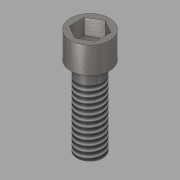
# Autodesk Inventor part: Bolt 2.0
Saved by Autodesk Inventor 2017 (Build 210142000, 142)
## iProperties
Created: 2017-01-01
Part Number: Bolt 2.0
Material: Steel, Galvanized
Document SubType Name: Modeling
Designer: qupec
Density: 7.85 g/cm^3
Appearance: Galvanized
Author: qupec
Autodesk Inventor part; units mm, degrees
ref_plane "YZ Plane" through (0, 0, 0) normal (1, 0, 0) x (0, 1, 0)
ref_plane "XZ Plane" through (0, 0, 0) normal (0, 1, 0) x (-1, 0, 0)
ref_plane "XY Plane" through (0, 0, 0) normal (0, 0, 1) x (1, 0, 0)
sketch "Sketch1" plane through (0, 0, 0) normal (0, 1, 0) x (-1, 0, 0)
  circle A0 centre (0, 0) radius 3.1369
  dimension "d0" = 6.2738
  constraints: 1 centre point, 1 coincident
  measures "d0" diameter of A0
extrude "Extrusion1" add sketch "Sketch1" along normal mid plane 6.35
sketch "Sketch2" plane through (0, 3.175, 0) normal (0, 1, 0) x (1, 0, 0)
  circle A0 centre (0, 0) radius 4.699
  dimension "d3" = 9.398
  constraints: 1 centre point, 1 coincident
  measures "d3" diameter of A0
extrude "Extrusion2" add sketch "Sketch2" along normal blind 6.35
sketch "Sketch3" plane through (0, -3.175, 0) normal (0, -1, 0) x (1, 0, 0)
  circle A0 centre (0, 0) radius 3.1369
  constraints: 1 centre point, 1 coincident
extrude "Extrusion3" add sketch "Sketch3" along normal blind 12.7
thread "Thread1" size "1/4-20 UNC" class "2A" standard "ANSI Unified Screw Threads" length 15.875
sketch "Sketch4" plane through (0, 9.525, 0) normal (0, 1, 0) x (1, 0, 0)
  line L0 (0, -3.6955) -> (-3.2004, -1.8478)
  line L1 (-3.2004, -1.8478) -> (-3.2004, 1.8478)
  line L2 (-3.2004, 1.8478) -> (0, 3.6955)
  line L3 (0, 3.6955) -> (3.2004, 1.8478)
  line L4 (3.2004, 1.8478) -> (3.2004, -1.8478)
  line L5 (3.2004, -1.8478) -> (0, -3.6955)
  point P0 (0, 0)
  point P1 (0, 0)
  dimension "d10" = 6.4008
  constraints: 12 end point, 1 coincident, 13 other
  measures "d10" distance between parallel lines of L1 L4
extrude "Extrusion4" cut sketch "Sketch4" against normal blind 3.81
body "Solid1"
